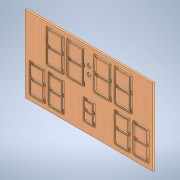
# Autodesk Inventor part: Schablone
Saved by Autodesk Inventor 2020 (Build 240168000, 168)
## iProperties
Created: 2023-11-19
Part Number: Schablone
Material: Holz (Kirsche)
Document SubType Name: Modeling
Designer: Schüle
Density: 0.63 g/cm^3
Appearance: Kirsche - natur - schwacher Glanz
Project: 7 Segment Anzeige
Description: Schablone ( A0)
Author: Schüle
Title: Spielstandsanzeige
Autodesk Inventor part; units mm, degrees
ref_plane "YZ Plane" through (0, 0, 0) normal (1, 0, 0) x (0, 1, 0)
ref_plane "XZ Plane" through (0, 0, 0) normal (0, 1, 0) x (-1, 0, 0)
ref_plane "XY Plane" through (0, 0, 0) normal (0, 0, 1) x (1, 0, 0)
sketch "Skizze1" plane through (0, 0, 0) normal (0, 0, 1) x (1, 0, 0)
  line L0 (-500, 300) -> (500, 300)
  line L1 (500, 300) -> (500, -300)
  line L2 (500, -300) -> (-500, -300)
  line L3 (-500, -300) -> (-500, 300)
  point P0 (0, 0)
  point P1 (0, 300)
  point P2 (500, 0)
  dimension "d0" = 1000
  dimension "d1" = 600
  constraints: 8 end point, 2 midpoint, 2 parallel, 1 horizontal, 1 horizontal alignment, 1 perpendicular, 1 vertical alignment
  measures "d0" distance of L1.end L2.end
  measures "d1" distance of L0.end L1.end
extrude "Grundplatte" add sketch "Skizze1" along normal blind 12
sketch "Skizze2" plane through (0, 0, 12) normal (0, 0, 1) x (1, 0, 0)
  line L0 (-334.3936, 270) -> (-314.3936, 250)
  line L1 (-314.3936, 250) -> (-219.3936, 250)
  line L2 (-219.3936, 250) -> (-199.3936, 270)
  line L3 (-199.3936, 270) -> (-334.3936, 270)
  line L4 (-209.3936, 260) -> (-205.8581, 256.4645) construction
  line L5 (-205.8581, 256.4645) -> (-195.8581, 266.4645)
  line L6 (-215.8581, 151.4645) -> (-215.8581, 246.4645)
  line L7 (-215.8581, 246.4645) -> (-205.8581, 256.4645)
  line L8 (-199.3936, 270) -> (-195.8581, 266.4645) construction
  line L9 (-219.3936, 250) -> (-215.8581, 246.4645) construction
  line L10 (-314.3936, 250) -> (-317.9291, 246.4645) construction
  line L11 (-317.9291, 246.4645) -> (-337.9291, 266.4645)
  line L12 (-337.9291, 266.4645) -> (-334.3936, 270) construction
  line L13 (-317.9291, 246.4645) -> (-317.9291, 151.4645)
  line L14 (-324.3936, 137.9289) -> (-314.3936, 147.9289)
  line L15 (-327.9291, 141.4645) -> (-337.9291, 141.4645)
  line L16 (-205.8581, 141.4645) -> (-195.8581, 141.4645)
  line L17 (-317.9291, 151.4645) -> (-327.9291, 141.4645)
  line L18 (-337.9291, 141.4645) -> (-337.9291, 266.4645)
  line L19 (-215.8581, 151.4645) -> (-205.8581, 141.4645)
  line L20 (-195.8581, 141.4645) -> (-195.8581, 266.4645)
  line L21 (-317.9291, 151.4645) -> (-314.3936, 147.9289) construction
  line L22 (-324.3936, 137.9289) -> (-327.9291, 141.4645) construction
  line L23 (-324.3936, 137.9289) -> (-314.3936, 127.9289)
  line L24 (-314.3936, 127.9289) -> (-219.3936, 127.9289)
  line L25 (-219.3936, 127.9289) -> (-209.3936, 137.9289)
  line L26 (-209.3936, 137.9289) -> (-219.3936, 147.9289)
  line L27 (-219.3936, 147.9289) -> (-314.3936, 147.9289)
  line L28 (-219.3936, 147.9289) -> (-215.8581, 151.4645) construction
  line L29 (-209.3936, 137.9289) -> (-205.8581, 141.4645) construction
  line L30 (-337.9291, 134.3934) -> (-337.9291, 9.3934)
  line L31 (-337.9291, 9.3934) -> (-317.9291, 29.3934)
  line L32 (-317.9291, 29.3934) -> (-317.9291, 124.3934)
  line L33 (-317.9291, 124.3934) -> (-327.9291, 134.3934)
  line L34 (-327.9291, 134.3934) -> (-337.9291, 134.3934)
  line L35 (-324.3936, 137.9289) -> (-327.9291, 134.3934) construction
  line L36 (-314.3936, 127.9289) -> (-317.9291, 124.3934) construction
  line L37 (-209.3936, 137.9289) -> (-205.8581, 134.3934) construction
  line L38 (-205.8581, 134.3934) -> (-215.8581, 124.3934)
  line L39 (-215.8581, 124.3934) -> (-219.3936, 127.9289) construction
  line L40 (-215.8581, 124.3934) -> (-215.8581, 29.3934)
  line L41 (-215.8581, 29.3934) -> (-195.8581, 9.3934)
  line L42 (-195.8581, 9.3934) -> (-195.8581, 134.3934)
  line L43 (-195.8581, 134.3934) -> (-205.8581, 134.3934)
  line L44 (-317.9291, 29.3934) -> (-314.3936, 25.8579) construction
  line L45 (-314.3936, 25.8579) -> (-334.3936, 5.8579)
  line L46 (-334.3936, 5.8579) -> (-337.9291, 9.3934) construction
  line L47 (-314.3936, 25.8579) -> (-219.3936, 25.8579)
  line L48 (-219.3936, 25.8579) -> (-215.8581, 29.3934) construction
  line L49 (-219.3936, 25.8579) -> (-199.3936, 5.8579)
  line L50 (-199.3936, 5.8579) -> (-195.8581, 9.3934) construction
  line L51 (-199.3936, 5.8579) -> (-334.3936, 5.8579)
  line L52 (-172.3225, 270) -> (-152.3225, 250)
  line L53 (-152.3225, 250) -> (-57.3225, 250)
  line L54 (-57.3225, 250) -> (-37.3225, 270)
  line L55 (-37.3225, 270) -> (-172.3225, 270)
  line L56 (-47.3225, 260) -> (-43.787, 256.4645) construction
  line L57 (-43.787, 256.4645) -> (-33.787, 266.4645)
  line L58 (-53.787, 151.4645) -> (-53.787, 246.4645)
  line L59 (-53.787, 246.4645) -> (-43.787, 256.4645)
  line L60 (-37.3225, 270) -> (-33.787, 266.4645) construction
  line L61 (-57.3225, 250) -> (-53.787, 246.4645) construction
  line L62 (-152.3225, 250) -> (-155.8581, 246.4645) construction
  line L63 (-155.8581, 246.4645) -> (-175.8581, 266.4645)
  line L64 (-175.8581, 266.4645) -> (-172.3225, 270) construction
  line L65 (-155.8581, 246.4645) -> (-155.8581, 151.4645)
  line L66 (-162.3225, 137.9289) -> (-152.3225, 147.9289)
  line L67 (-165.8581, 141.4645) -> (-175.8581, 141.4645)
  line L68 (-43.787, 141.4645) -> (-33.787, 141.4645)
  line L69 (-155.8581, 151.4645) -> (-165.8581, 141.4645)
  line L70 (-175.8581, 141.4645) -> (-175.8581, 266.4645)
  line L71 (-53.787, 151.4645) -> (-43.787, 141.4645)
  line L72 (-33.787, 141.4645) -> (-33.787, 266.4645)
  line L73 (-155.8581, 151.4645) -> (-152.3225, 147.9289) construction
  line L74 (-162.3225, 137.9289) -> (-165.8581, 141.4645) construction
  line L75 (-162.3225, 137.9289) -> (-152.3225, 127.9289)
  line L76 (-152.3225, 127.9289) -> (-57.3225, 127.9289)
  line L77 (-57.3225, 127.9289) -> (-47.3225, 137.9289)
  line L78 (-47.3225, 137.9289) -> (-57.3225, 147.9289)
  line L79 (-57.3225, 147.9289) -> (-152.3225, 147.9289)
  line L80 (-57.3225, 147.9289) -> (-53.787, 151.4645) construction
  line L81 (-47.3225, 137.9289) -> (-43.787, 141.4645) construction
  line L82 (-175.8581, 134.3934) -> (-175.8581, 9.3934)
  line L83 (-175.8581, 9.3934) -> (-155.8581, 29.3934)
  line L84 (-155.8581, 29.3934) -> (-155.8581, 124.3934)
  line L85 (-155.8581, 124.3934) -> (-165.8581, 134.3934)
  line L86 (-165.8581, 134.3934) -> (-175.8581, 134.3934)
  line L87 (-162.3225, 137.9289) -> (-165.8581, 134.3934) construction
  line L88 (-152.3225, 127.9289) -> (-155.8581, 124.3934) construction
  line L89 (-47.3225, 137.9289) -> (-43.787, 134.3934) construction
  line L90 (-43.787, 134.3934) -> (-53.787, 124.3934)
  line L91 (-53.787, 124.3934) -> (-57.3225, 127.9289) construction
  line L92 (-53.787, 124.3934) -> (-53.787, 29.3934)
  line L93 (-53.787, 29.3934) -> (-33.787, 9.3934)
  line L94 (-33.787, 9.3934) -> (-33.787, 134.3934)
  line L95 (-33.787, 134.3934) -> (-43.787, 134.3934)
  line L96 (-155.8581, 29.3934) -> (-152.3225, 25.8579) construction
  line L97 (-152.3225, 25.8579) -> (-172.3225, 5.8579)
  line L98 (-172.3225, 5.8579) -> (-175.8581, 9.3934) construction
  line L99 (-152.3225, 25.8579) -> (-57.3225, 25.8579)
  line L100 (-57.3225, 25.8579) -> (-53.787, 29.3934) construction
  line L101 (-57.3225, 25.8579) -> (-37.3225, 5.8579)
  line L102 (-37.3225, 5.8579) -> (-33.787, 9.3934) construction
  line L103 (-37.3225, 5.8579) -> (-172.3225, 5.8579)
  line L104 (500, 300) -> (-500, 300) projected
  line L105 (0, 300) -> (0, -300) construction
  line L106 (-500, -300) -> (500, -300) projected
  point P0 (-327.9291, 256.4645)
  point P1 (-165.8581, 256.4645)
  dimension "d5" = 5
  dimension "d6" = 45
  dimension "d7" = 20
  dimension "d13" = 5
  dimension "d14" = 115
  dimension "d15" = 115
  dimension "d16" = 5
  dimension "d17" = 45
  dimension "d18" = 20
  dimension "d19" = 5
  dimension "d20" = 115
  dimension "d21" = 115
  dimension "d39" = 20
  dimension "d41" = 30
  dimension "d42" = 67.574
  constraints: 212 end point, 50 perpendicular, 24 equal length, 24 parallel, 8 vertical, 6 horizontal, 6 midpoint, 6 point on line, 6 vertical alignment, 5 horizontal alignment, 2 collinear
  measures "d5" distance of L2.end L5.end
  measures "d6" angle of L3 L2
  measures "d7" distance between parallel lines of L1 L3
  measures "d13" distance of L13.end L14.end
  measures "d14" distance of L25.end L14.start
  measures "d15" distance of L4.end L16.start
  measures "d16" distance of L55.start L60.end
  measures "d17" angle of L55 L54
  measures "d18" distance between parallel lines of L53 L55
  measures "d19" distance of L65.end L66.end
  measures "d20" distance of L78.start L66.start
  measures "d21" distance of L59.end L71.end
  measures "d39" distance between parallel lines of L42 L82
  measures "d41" distance between parallel lines of L104 L55
  measures "d42" diameter of L72 L105
extrude "Minutenanzeige" cut sketch "Skizze2" against normal through all
mirror "Sekundenanzeige" about plane through (0, 0, 0) normal (1, 0, 0) of "Minutenanzeige"
sketch "Skizze3" plane through (0, 0, 12) normal (0, 0, 1) x (1, 0, 0)
  line L0 (-43, -64) -> (43, -64)
  line L1 (43, -64) -> (23, -84)
  line L2 (23, -84) -> (-23, -84)
  line L3 (-23, -84) -> (-43, -64)
  line L4 (-43, -64) -> (-46.5355, -67.5355) construction
  line L5 (-46.5355, -67.5355) -> (-26.5355, -87.5355)
  line L6 (-26.5355, -87.5355) -> (-23, -84) construction
  line L7 (-46.5355, -67.5355) -> (-46.5355, -143.5355)
  line L8 (-46.5355, -143.5355) -> (-36.5355, -143.5355)
  line L9 (-36.5355, -143.5355) -> (-26.5355, -133.5355)
  line L10 (-26.5355, -133.5355) -> (-26.5355, -87.5355)
  line L11 (43, -64) -> (46.5355, -67.5355) construction
  line L12 (46.5355, -67.5355) -> (26.5355, -87.5355)
  line L13 (26.5355, -87.5355) -> (23, -84) construction
  line L14 (26.5355, -87.5355) -> (26.5355, -133.5355)
  line L15 (26.5355, -133.5355) -> (36.5355, -143.5355)
  line L16 (36.5355, -143.5355) -> (46.5355, -143.5355)
  line L17 (46.5355, -143.5355) -> (46.5355, -67.5355)
  line L18 (-26.5355, -133.5355) -> (-23, -137.0711) construction
  line L19 (-23, -137.0711) -> (-33, -147.0711)
  line L20 (-33, -147.0711) -> (-36.5355, -143.5355) construction
  line L21 (-33, -147.0711) -> (-23, -157.0711)
  line L22 (-23, -137.0711) -> (23, -137.0711)
  line L23 (23, -137.0711) -> (26.5355, -133.5355) construction
  line L24 (23, -137.0711) -> (33, -147.0711)
  line L25 (33, -147.0711) -> (36.5355, -143.5355) construction
  line L26 (33, -147.0711) -> (23, -157.0711)
  line L27 (23, -157.0711) -> (-23, -157.0711)
  line L28 (-46.5355, -150.6066) -> (-46.5355, -226.6066)
  line L29 (-46.5355, -226.6066) -> (-26.5355, -206.6066)
  line L30 (-26.5355, -206.6066) -> (-26.5355, -160.6066)
  line L31 (-26.5355, -160.6066) -> (-36.5355, -150.6066)
  line L32 (-36.5355, -150.6066) -> (-46.5355, -150.6066)
  line L33 (-33, -147.0711) -> (-36.5355, -150.6066) construction
  line L34 (-26.5355, -160.6066) -> (-23, -157.0711) construction
  line L35 (-46.5355, -226.6066) -> (-43, -230.1421) construction
  line L36 (-43, -230.1421) -> (-23, -210.1421)
  line L37 (-23, -210.1421) -> (-26.5355, -206.6066) construction
  line L38 (-23, -210.1421) -> (23, -210.1421)
  line L39 (23, -210.1421) -> (43, -230.1421)
  line L40 (43, -230.1421) -> (-43, -230.1421)
  line L41 (23, -210.1421) -> (26.5355, -206.6066) construction
  line L42 (26.5355, -206.6066) -> (46.5355, -226.6066)
  line L43 (46.5355, -226.6066) -> (43, -230.1421) construction
  line L44 (26.5355, -206.6066) -> (26.5355, -160.6066)
  line L45 (26.5355, -160.6066) -> (23, -157.0711) construction
  line L46 (26.5355, -160.6066) -> (36.5355, -150.6066)
  line L47 (36.5355, -150.6066) -> (46.5355, -150.6066)
  line L48 (46.5355, -150.6066) -> (46.5355, -226.6066)
  line L49 (33, -147.0711) -> (36.5355, -150.6066) construction
  line L50 (-37.3225, 5.8579) -> (-172.3225, 5.8579) projected
  line L51 (172.3225, 5.8579) -> (37.3225, 5.8579) projected
  line L52 (-57.3225, 25.8579) -> (-37.3225, 5.8579) projected
  line L53 (-37.3225, 5.8579) -> (37.3225, 5.8579) construction
  line L54 (0, 5.8579) -> (0, -300) construction
  line L55 (-500, -300) -> (500, -300) projected
  line L56 (-33, -147.0711) -> (33, -147.0711) construction
  point P0 (0, 0)
  point P1 (36.5355, -77.5355)
  point P2 (0, -84)
  point P3 (0, -147.0711)
  dimension "d45" = 45
  dimension "d46" = 66
  dimension "d47" = 5
  dimension "d48" = 66
  dimension "d49" = 20
  dimension "d50" = 20
  constraints: 107 end point, 29 perpendicular, 10 equal length, 8 parallel, 6 midpoint, 6 vertical, 3 horizontal, 3 vertical alignment, 1 horizontal alignment, 1 point on line
  measures "d45" angle of L0 L1
  measures "d46" distance of L24.end L19.end
  measures "d47" distance of L9.end L18.end
  measures "d48" distance from line of L16 point (36.536, -77.536)
  measures "d49" distance between parallel lines of L27 L22
  measures "d50" distance between parallel lines of L0 L2
extrude "Halbzeit" cut sketch "Skizze3" against normal through all
sketch "Skizze4" plane through (0, 0, 12) normal (0, 0, 1) x (1, 0, 0)
  line L0 (-466.4645, -30) -> (-346.4645, -30)
  line L1 (-346.4645, -30) -> (-366.4645, -50)
  line L2 (-366.4645, -50) -> (-446.4645, -50)
  line L3 (-446.4645, -50) -> (-466.4645, -30)
  line L4 (-466.4645, -30) -> (-470, -33.5355) construction
  line L5 (-470, -33.5355) -> (-450, -53.5355)
  line L6 (-450, -53.5355) -> (-446.4645, -50) construction
  line L7 (-346.4645, -30) -> (-342.9289, -33.5355) construction
  line L8 (-342.9289, -33.5355) -> (-362.9289, -53.5355)
  line L9 (-362.9289, -53.5355) -> (-366.4645, -50) construction
  line L10 (-362.9289, -53.5355) -> (-362.9289, -133.5355)
  line L11 (-362.9289, -133.5355) -> (-352.9289, -143.5355)
  line L12 (-352.9289, -143.5355) -> (-342.9289, -143.5355)
  line L13 (-342.9289, -143.5355) -> (-342.9289, -33.5355)
  line L14 (-362.9289, -133.5355) -> (-366.4645, -137.0711) construction
  line L15 (-366.4645, -137.0711) -> (-356.4645, -147.0711)
  line L16 (-356.4645, -147.0711) -> (-352.9289, -143.5355) construction
  line L17 (-450, -53.5355) -> (-450, -133.5355)
  line L18 (-450, -133.5355) -> (-460, -143.5355)
  line L19 (-460, -143.5355) -> (-470, -143.5355)
  line L20 (-470, -143.5355) -> (-470, -33.5355)
  line L21 (-450, -133.5355) -> (-446.4645, -137.0711) construction
  line L22 (-446.4645, -137.0711) -> (-456.4645, -147.0711)
  line L23 (-456.4645, -147.0711) -> (-460, -143.5355) construction
  line L24 (-446.4645, -137.0711) -> (-366.4645, -137.0711)
  line L25 (-456.4645, -147.0711) -> (-446.4645, -157.0711)
  line L26 (-446.4645, -157.0711) -> (-366.4645, -157.0711)
  line L27 (-366.4645, -157.0711) -> (-356.4645, -147.0711)
  line L28 (-456.4645, -147.0711) -> (-460, -150.6066) construction
  line L29 (-460, -150.6066) -> (-450, -160.6066)
  line L30 (-450, -160.6066) -> (-446.4645, -157.0711) construction
  line L31 (-366.4645, -157.0711) -> (-362.9289, -160.6066) construction
  line L32 (-362.9289, -160.6066) -> (-352.9289, -150.6066)
  line L33 (-352.9289, -150.6066) -> (-356.4645, -147.0711) construction
  line L34 (-460, -150.6066) -> (-470, -150.6066)
  line L35 (-470, -150.6066) -> (-470, -260.6066)
  line L36 (-470, -260.6066) -> (-450, -240.6066)
  line L37 (-450, -240.6066) -> (-450, -160.6066)
  line L38 (-352.9289, -150.6066) -> (-342.9289, -150.6066)
  line L39 (-342.9289, -150.6066) -> (-342.9289, -260.6066)
  line L40 (-342.9289, -260.6066) -> (-362.9289, -240.6066)
  line L41 (-362.9289, -240.6066) -> (-362.9289, -160.6066)
  line L42 (-450, -240.6066) -> (-446.4645, -244.1421) construction
  line L43 (-446.4645, -244.1421) -> (-466.4645, -264.1421)
  line L44 (-466.4645, -264.1421) -> (-470, -260.6066) construction
  line L45 (-362.9289, -240.6066) -> (-366.4645, -244.1421) construction
  line L46 (-366.4645, -244.1421) -> (-346.4645, -264.1421)
  line L47 (-346.4645, -264.1421) -> (-342.9289, -260.6066) construction
  line L48 (-366.4645, -244.1421) -> (-446.4645, -244.1421)
  line L49 (-466.4645, -264.1421) -> (-346.4645, -264.1421)
  line L50 (-319.3934, -30) -> (-199.3934, -30)
  line L51 (-199.3934, -30) -> (-219.3934, -50)
  line L52 (-219.3934, -50) -> (-299.3934, -50)
  line L53 (-299.3934, -50) -> (-319.3934, -30)
  line L54 (-319.3934, -30) -> (-322.9289, -33.5355) construction
  line L55 (-322.9289, -33.5355) -> (-302.9289, -53.5355)
  line L56 (-302.9289, -53.5355) -> (-299.3934, -50) construction
  line L57 (-199.3934, -30) -> (-195.8579, -33.5355) construction
  line L58 (-195.8579, -33.5355) -> (-215.8579, -53.5355)
  line L59 (-215.8579, -53.5355) -> (-219.3934, -50) construction
  line L60 (-215.8579, -53.5355) -> (-215.8579, -133.5355)
  line L61 (-215.8579, -133.5355) -> (-205.8579, -143.5355)
  line L62 (-205.8579, -143.5355) -> (-195.8579, -143.5355)
  line L63 (-195.8579, -143.5355) -> (-195.8579, -33.5355)
  line L64 (-215.8579, -133.5355) -> (-219.3934, -137.0711) construction
  line L65 (-219.3934, -137.0711) -> (-209.3934, -147.0711)
  line L66 (-209.3934, -147.0711) -> (-205.8579, -143.5355) construction
  line L67 (-302.9289, -53.5355) -> (-302.9289, -133.5355)
  line L68 (-302.9289, -133.5355) -> (-312.9289, -143.5355)
  line L69 (-312.9289, -143.5355) -> (-322.9289, -143.5355)
  line L70 (-322.9289, -143.5355) -> (-322.9289, -33.5355)
  line L71 (-302.9289, -133.5355) -> (-299.3934, -137.0711) construction
  line L72 (-299.3934, -137.0711) -> (-309.3934, -147.0711)
  line L73 (-309.3934, -147.0711) -> (-312.9289, -143.5355) construction
  line L74 (-299.3934, -137.0711) -> (-219.3934, -137.0711)
  line L75 (-309.3934, -147.0711) -> (-299.3934, -157.0711)
  line L76 (-299.3934, -157.0711) -> (-219.3934, -157.0711)
  line L77 (-219.3934, -157.0711) -> (-209.3934, -147.0711)
  line L78 (-309.3934, -147.0711) -> (-312.9289, -150.6066) construction
  line L79 (-312.9289, -150.6066) -> (-302.9289, -160.6066)
  line L80 (-302.9289, -160.6066) -> (-299.3934, -157.0711) construction
  line L81 (-219.3934, -157.0711) -> (-215.8579, -160.6066) construction
  line L82 (-215.8579, -160.6066) -> (-205.8579, -150.6066)
  line L83 (-205.8579, -150.6066) -> (-209.3934, -147.0711) construction
  line L84 (-312.9289, -150.6066) -> (-322.9289, -150.6066)
  line L85 (-322.9289, -150.6066) -> (-322.9289, -260.6066)
  line L86 (-322.9289, -260.6066) -> (-302.9289, -240.6066)
  line L87 (-302.9289, -240.6066) -> (-302.9289, -160.6066)
  line L88 (-205.8579, -150.6066) -> (-195.8579, -150.6066)
  line L89 (-195.8579, -150.6066) -> (-195.8579, -260.6066)
  line L90 (-195.8579, -260.6066) -> (-215.8579, -240.6066)
  line L91 (-215.8579, -240.6066) -> (-215.8579, -160.6066)
  line L92 (-302.9289, -240.6066) -> (-299.3934, -244.1421) construction
  line L93 (-299.3934, -244.1421) -> (-319.3934, -264.1421)
  line L94 (-319.3934, -264.1421) -> (-322.9289, -260.6066) construction
  line L95 (-215.8579, -240.6066) -> (-219.3934, -244.1421) construction
  line L96 (-219.3934, -244.1421) -> (-199.3934, -264.1421)
  line L97 (-199.3934, -264.1421) -> (-195.8579, -260.6066) construction
  line L98 (-219.3934, -244.1421) -> (-299.3934, -244.1421)
  line L99 (-319.3934, -264.1421) -> (-199.3934, -264.1421)
  line L100 (-199.3936, 5.8579) -> (-334.3936, 5.8579) projected
  line L101 (-500, -300) -> (500, -300) projected
  line L102 (-46.5355, -143.5355) -> (-46.5355, -67.5355) projected
  line L103 (-46.5355, -226.6066) -> (-46.5355, -150.6066) projected
  line L104 (-500, 300) -> (-500, -300) projected
  line L105 (-46.5355, -150.6066) -> (-36.5355, -150.6066) projected
  line L106 (-46.5355, -143.5355) -> (-46.5355, -150.6066) construction
  line L107 (-46.5355, -147.0711) -> (-500, -147.0711) construction
  line L108 (-500, 300) -> (-500, -300) projected
  line L109 (-356.4645, -147.0711) -> (-309.3934, -147.0711) construction
  point P0 (0, 0)
  point P1 (-352.9289, -43.5355)
  point P2 (-205.8579, -43.5355)
  dimension "d53" = 45
  dimension "d54" = 20
  dimension "d55" = 5
  dimension "d56" = 20
  dimension "d57" = 100
  dimension "d58" = 100
  dimension "d59" = 45
  dimension "d60" = 20
  dimension "d61" = 5
  dimension "d62" = 20
  dimension "d63" = 100
  dimension "d64" = 100
  dimension "d65" = 20
  dimension "d72" = 30
  constraints: 206 end point, 57 perpendicular, 32 equal length, 12 horizontal, 8 parallel, 7 vertical, 4 vertical alignment, 3 midpoint, 3 point on line, 2 horizontal alignment
  measures "d53" angle of L1 L0
  measures "d54" distance between parallel lines of L2 L0
  measures "d55" distance of L0.start L4.end
  measures "d56" distance between parallel lines of L26 L24
  measures "d57" distance of L15.end L22.end
  measures "d58" distance from line of point (-352.929, -43.536) L12
  measures "d59" angle of L51 L50
  measures "d60" distance between parallel lines of L52 L50
  measures "d61" distance of L50.start L54.end
  measures "d62" distance between parallel lines of L76 L74
  measures "d63" distance of L65.end L72.end
  measures "d64" distance from line of point (-205.858, -43.536) L62
  measures "d65" distance between parallel lines of L70 L13
  measures "d72" distance between parallel lines of L104 L20
extrude "Spielstand_Heim" cut sketch "Skizze4" against normal through all
sketch "Skizze5" plane through (0, 0, 12) normal (0, 0, 1) x (1, 0, 0)
  line L0 (-33.787, 266.4645) -> (-33.787, 141.4645) projected
  line L1 (-33.787, 134.3934) -> (-33.787, 9.3934) projected
  line L2 (33.787, 141.4645) -> (33.787, 266.4645) projected
  line L3 (33.787, 9.3934) -> (33.787, 134.3934) projected
  line L4 (-57.3225, 147.9289) -> (-47.3225, 137.9289) projected
  line L5 (47.3225, 137.9289) -> (57.3225, 147.9289) projected
  line L6 (-47.3225, 137.9289) -> (47.3225, 137.9289) construction
  line L7 (0, 137.9289) -> (0, 167.9289) construction
  line L8 (0, 137.9289) -> (0, 107.9289) construction
  circle A0 centre (0, 167.9289) radius 15
  circle A1 centre (0, 107.9289) radius 15
  point P0 (0, 0)
  dimension "d68" = 30
  dimension "d69" = 30
  constraints: 6 end point, 2 centre point, 2 coincident, 2 vertical, 1 collinear, 1 equal radius, 1 horizontal, 1 midpoint
  measures "d68" diameter of A0
  measures "d69" distance of L7.start L7.end
mirror "Spielstand_Gast" about plane through (0, 0, 0) normal (1, 0, 0) of "Spielstand_Heim"
extrude "Extrusion5" cut sketch "Skizze5" against normal through all
